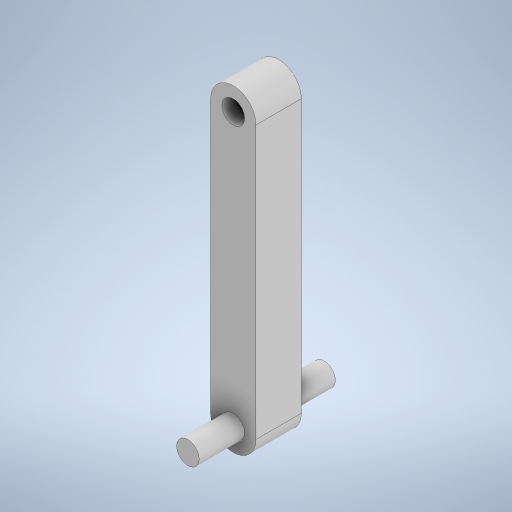
# Autodesk Inventor part: arm1
Saved by Autodesk Inventor 2024 (Build 280153000, 153)
## iProperties
Created: 2024-08-23
Part Number: arm1
Material: Generic
Document SubType Name: Modeling
Designer: domko
Density: 1 g/cm^3
Appearance: Default
Author: domko
Autodesk Inventor part; units mm, degrees
ref_plane "YZ Plane" through (0, 0, 0) normal (1, 0, 0) x (0, 1, 0)
ref_plane "XZ Plane" through (0, 0, 0) normal (0, 1, 0) x (-1, 0, 0)
ref_plane "XY Plane" through (0, 0, 0) normal (0, 0, 1) x (1, 0, 0)
sketch "Sketch1" plane through (0, 0, 0) normal (0, 0, 1) x (1, 0, 0)
  line L0 (10, 99.1499) -> (10, -20.8501)
  line L1 (-10, -20.8501) -> (-10, 99.1499)
  arc A0 (-10, -20.8501) -> (10, -20.8501) centre (0, -20.8501) ccw
  arc A1 (10, 99.1499) -> (-10, 99.1499) centre (0, 99.1499) ccw
  circle A2 centre (0, 99.1499) radius 5
  point P0 (0, 0)
  dimension "d0" = 10
  dimension "d1" = 20
  dimension "d2" = 120
  dimension "d3" = 10
  constraints: 4 end point, 4 point on circle, 4 tangent, 3 centre point, 1 coincident, 1 parallel
  measures "d0" distance from line of point (0, 0) L1
  measures "d1" distance between parallel lines of L0 L1
  measures "d2" distance of L0.start L0.end
  measures "d3" diameter of A2
extrude "Extrusion1" add sketch "Sketch1" along normal blind 20
sketch "Sketch2" plane through (0, 0, 20) normal (0, 0, 1) x (1, 0, 0)
  arc A0 (-10, -20.8501) -> (10, -20.8501) centre (0, -20.8501) ccw projected
  circle A1 centre (0, -20.8501) radius 5
  point P0 (0, 0)
  point P1 (0, -20.8501)
  point P2 (0, -30.8501)
  dimension "d7" = 10
  dimension "d8" = 10
  constraints: 1 centre point, 1 coincident, 1 point on circle
  measures "d7" distance of point (0, -30.85) point (0, -20.85)
  measures "d8" diameter of A1
extrude "Extrusion2" add sketch "Sketch2" along normal blind 20 and the other way blind 40
body "Solid1"
